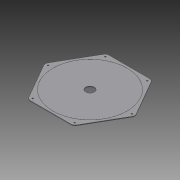
# Autodesk Inventor part: Heatbed_170mm_Hex
Saved by Autodesk Inventor 2014 (Build 180170000, 170)
## iProperties
Created: 2014-11-03
Part Number: Heatbed_170mm_Hex
Material: Generic
Document SubType Name: Modeling
Designer: ThatOtherGuy
Density: 1 g/cm^3
Appearance: Default
Author: ThatOtherGuy
Autodesk Inventor part; units mm, degrees
ref_plane "YZ Plane" through (0, 0, 0) normal (1, 0, 0) x (0, 1, 0)
ref_plane "XZ Plane" through (0, 0, 0) normal (0, 1, 0) x (-1, 0, 0)
ref_plane "XY Plane" through (0, 0, 0) normal (0, 0, 1) x (1, 0, 0)
sketch "Sketch1" plane through (0, 0, 0) normal (0, 0, 1) x (1, 0, 0)
  line L0 (51.9615, 90) -> (103.923, 0)
  line L1 (103.923, 0) -> (51.9615, -90)
  line L2 (51.9615, -90) -> (-51.9615, -90)
  line L3 (-51.9615, -90) -> (-103.923, 0)
  line L4 (-103.923, 0) -> (-51.9615, 90)
  line L5 (-51.9615, 90) -> (51.9615, 90)
  circle A0 centre (0, 0) radius 85
  circle A1 centre (0, 0) radius 10
  dimension "d1" = 170
  dimension "d2" = 180
  dimension "d12" = 20
  constraints: 12 end point, 3 coincident, 2 centre point, 1 horizontal, 13 other
  measures "d1" diameter of A0
  measures "d2" distance between parallel lines of L2 L5
  measures "d12" diameter of A1
extrude "Extrusion1" add sketch "Sketch1" along normal blind 1.6 contours L0 L1 L2 L3 L4 L5 | A0
sketch "Sketch3" plane through (0, 0, 1.6) normal (0, 0, 1) x (1, 0, 0)
  circle A0 centre (0, 0) radius 10 projected
  circle A1 centre (-96, 0) radius 1.6
  line L0 (-51.9615, 90) -> (-103.923, 0) projected
  line L1 (-103.923, 0) -> (-51.9615, -90) projected
  arc A2 (-101.2676, 4.5994) -> (-101.2676, -4.5994) centre (-93.3013, 0) ccw
  dimension "d13" = 96
  dimension "d14" = 3.2
  dimension "d20" = 9.1987
  dimension "d21" = 93.3013
  constraints: 2 centre point, 2 point on circle, 2 point on line, 2 tangent, 1 horizontal alignment
  measures "d13" distance of A0.centre A1.centre
  measures "d14" diameter of A1
  measures "d20" radius of A2
  measures "d21" distance of A0.centre A2.centre
extrude "Extrusion3" cut sketch "Sketch3" against normal up to next contours A1 | A2 L1 L0
pattern_circular "Circular Pattern1" count 6 over 360 about axis through (0, 0, 0) along (0, 0, 1) of "Extrusion3"
sketch "Sketch4" plane through (0, 0, 1.6) normal (0, 0, 1) x (1, 0, 0)
  circle A0 centre (0, 0) radius 10 projected
  circle A1 centre (0, 0) radius 85
  dimension "d22" = 170
  constraints: 1 centre point, 1 coincident
  measures "d22" diameter of A1
extrude "Extrusion4" add sketch "Sketch4" along normal blind 0.1
body "Solid1"
